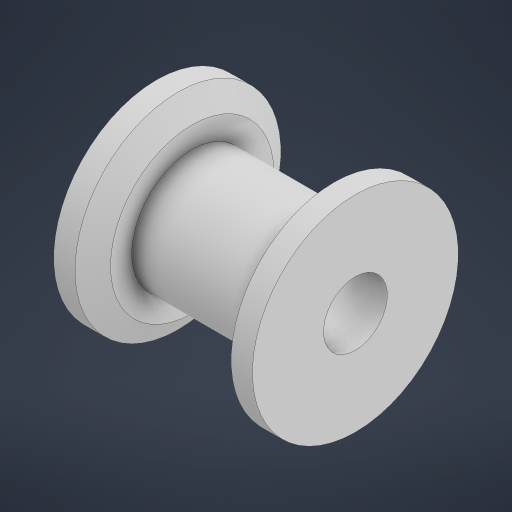
# Autodesk Inventor part: Hülse zum einhaken
Saved by Autodesk Inventor 2024.2 (Build 282272000, 272)
## iProperties
Created: 2023-12-02
Part Number: Hülse zum einhaken
Material: Generisch
Document SubType Name: Modeling
Designer: jacob
Density: 1 g/cm^3
Appearance: Vorgabe
Author: jacob
Autodesk Inventor part; units mm, degrees
ref_plane "YZ Plane" through (0, 0, 0) normal (1, 0, 0) x (0, 1, 0)
ref_plane "XZ Plane" through (0, 0, 0) normal (0, 1, 0) x (-1, 0, 0)
ref_plane "XY Plane" through (0, 0, 0) normal (0, 0, 1) x (1, 0, 0)
sketch "Skizze1" plane through (0, 0, 0) normal (0, 0, 1) x (1, 0, 0)
  line L0 (0, 0) -> (14, 0)
  line L1 (0, 2.25) -> (14, 2.25)
  line L2 (14, 2.25) -> (14, 7.25)
  line L3 (14, 7.25) -> (11.5, 7.25)
  line L4 (11.5, 7.25) -> (11.5, 4.25)
  line L5 (11.5, 4.25) -> (2.5, 4.25)
  line L6 (2.5, 4.25) -> (2.5, 7.25)
  line L7 (2.5, 7.25) -> (0, 7.25)
  line L8 (0, 7.25) -> (0, 2.25)
  dimension "d0" = 14
  dimension "d1" = 4.5
  dimension "d2" = 2
  dimension "d3" = 3
  dimension "d4" = 3
  dimension "d5" = 9
  constraints: 18 end point, 5 perpendicular, 3 horizontal, 2 vertical alignment, 1 collinear, 1 vertical
  measures "d0" distance of L0.start L0.end
  measures "d1" diameter of L1 L0
  measures "d2" distance between parallel lines of L5 L1
  measures "d3" distance of L3.end L4.end
  measures "d4" distance of L5.end L6.end
  measures "d5" distance of L4.end L5.end
revolve "Umdrehung1" add sketch "Skizze1" angle 360 about axis through (0, 0, 0) along (1, 0, 0)
chamfer "Fasen2" distance 1.5 distance2 1 1 edges at (2.5, -7.25, 0) measured on face at (2.5, 6.1798, -0.5783)
chamfer "Fasen3" distance 1 distance2 1.5 1 edges at (11.5, -7.25, 0) measured on face at (13.1667, 7.1561, -1.163)
